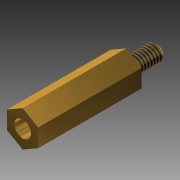
# Autodesk Inventor part: Standoff 40
Saved by Autodesk Inventor 2015 (Build 190159000, 159)
## iProperties
Created: 2016-02-18
Part Number: Standoff 40
Material: Brass
Document SubType Name: Modeling
Designer: 23902
Density: 8.49 g/cm^3
Appearance: Brass - Polished
Mass: 1.03642 g
Surface Area: 12.7978 cm^2
Volume: 0.925377 cm^3
Author: 23902
Autodesk Inventor part; units mm, degrees
ref_plane "YZ Plane" through (0, 0, 0) normal (1, 0, 0) x (0, 1, 0)
ref_plane "XZ Plane" through (0, 0, 0) normal (0, 1, 0) x (-1, 0, 0)
ref_plane "XY Plane" through (0, 0, 0) normal (0, 0, 1) x (1, 0, 0)
sketch "Sketch1" plane through (0, 0, 0) normal (0, 1, 0) x (-1, 0, 0)
  circle A0 centre (0, 0) radius 1.6
  line L0 (0, -3.4641) -> (-3, -1.7321)
  line L1 (-3, -1.7321) -> (-3, 1.7321)
  line L2 (-3, 1.7321) -> (0, 3.4641)
  line L3 (0, 3.4641) -> (3, 1.7321)
  line L4 (3, 1.7321) -> (3, -1.7321)
  line L5 (3, -1.7321) -> (0, -3.4641)
  dimension "d0" = 3.2
  dimension "d1" = 6
  constraints: 12 end point, 2 coincident, 1 centre point, 13 other
  measures "d0" diameter of A0
  measures "d1" distance between parallel lines of L0 L3
extrude "Extrusion1" add sketch "Sketch1" along normal blind 20
sketch "Sketch2" plane through (0, 20, 0) normal (0, 1, 0) x (1, 0, 0)
  circle A0 centre (0, 0) radius 1.6 projected
  line L0 (3, 1.7321) -> (0, 3.4641) projected
  line L1 (0, 3.4641) -> (-3, 1.7321) projected
  line L2 (-3, 1.7321) -> (-3, -1.7321) projected
  line L3 (-3, -1.7321) -> (0, -3.4641) projected
  line L4 (0, -3.4641) -> (3, -1.7321) projected
  line L5 (3, -1.7321) -> (3, 1.7321) projected
extrude "Extrusion2" add sketch "Sketch2" along normal blind 6 contours A0
chamfer "Chamfer1" distance 0.5 angle 45 1 edges at (-1.6, 26, 0)
thread "Thread1" size "M3.5x0.6" class "6g" standard "ANSI Metric M Profile" full length
body "Solid1"
